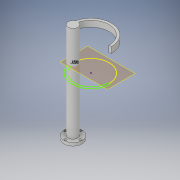
# Autodesk Inventor part: pincherleft
Saved by Autodesk Inventor 2017 (Build 210142000, 142)
## iProperties
Created: 2017-11-18
Part Number: pincherleft
Material: Generic
Document SubType Name: Modeling
Designer: User
Density: 1 g/cm^3
Appearance: Default
Author: User
Autodesk Inventor part; units mm, degrees
ref_plane "YZ Plane" through (0, 0, 0) normal (1, 0, 0) x (0, 1, 0)
ref_plane "XZ Plane" through (0, 0, 0) normal (0, 1, 0) x (-1, 0, 0)
ref_plane "XY Plane" through (0, 0, 0) normal (0, 0, 1) x (1, 0, 0)
sketch "Sketch1" plane through (0, 0, 0) normal (0, 1, 0) x (-1, 0, 0)
  circle A0 centre (0, 0) radius 5.08
  dimension "d0" = 10.16
  constraints: 1 centre point, 1 coincident
  measures "d0" diameter of A0
extrude "Extrusion1" add sketch "Sketch1" along normal blind 101.6
sketch "Sketch2" plane through (0, 101.6, 0) normal (0, 1, 0) x (1, 0, 0)
  circle A0 centre (0, 0) radius 5.08 projected
  line L0 (0, 0) -> (-2.54, 0)
  line L1 (38.1, 0) -> (40.64, 0)
  arc A1 (38.1, 0) -> (0, 0) centre (19.05, 0) ccw
  arc A2 (40.64, 0) -> (-2.54, 0) centre (19.05, 0) ccw
  line L2 (38.1, 0) -> (40.64, 0) construction
  line L3 (5.08, 0) -> (-2.54, 0) construction
  line L4 (-2.54, 0) -> (5.08, 0)
  line L5 (38.1, 0) -> (40.64, 0)
  dimension "d64" = 2.54
  dimension "d65" = 2.54
  dimension "d66" = 38.1
  dimension "d67" = 19.05
  dimension "d68" = 180
  dimension "d69" = 21.59
  constraints: 12 end point, 4 point on circle, 2 centre point, 2 coincident, 2 horizontal, 1 horizontal alignment, 1 other
  measures "d64" distance of L0.start L0.end
  measures "d65" distance of L1.start L1.end
  measures "d66" distance of L1.start L0.start
  measures "d67" distance of L1.start point (19.05, 0)
  measures "d68" angle of L3 L2
  measures "d69" distance of A2.centre L1.end
extrude "Extrusion5" add sketch "Sketch2" against normal blind 6.35 contours A1 L0 A2 A0 | A0 A2 L1 A1
sketch "Sketch4" plane through (0, 0, 0) normal (0, -1, 0) x (1, 0, 0)
  circle A0 centre (0, 0) radius 9.525
  dimension "d72" = 19.05
  constraints: 1 centre point, 1 coincident
  measures "d72" diameter of A0
extrude "Extrusion6" add sketch "Sketch4" along normal blind 3.175
sketch "Sketch5" plane through (0, -3.175, 0) normal (0, -1, 0) x (1, 0, 0)
  point P0 (0, 0)
  point P1 (0, 8.001)
  point P2 (0, -8.001)
  point P3 (8.001, 0)
  point P4 (-8.001, 0)
  dimension "d79" = 8.001
  dimension "d80" = 8.001
  dimension "d81" = 8.001
  dimension "d82" = 8.001
  measures "d79" distance of point (0, 0) point (0, 8.001)
  measures "d80" distance of point (0, 0) point (0, -8.001)
  measures "d81" distance of point (-8.001, 0) point (0, 0)
  measures "d82" distance of point (0, 0) point (8.001, 0)
hole "Hole1" at (0, -3.175, 8.001) at (0, -3.175, -8.001) at (8.001, -3.175, 0) at (-8.001, -3.175, 0) direction (0, 1, 0) diameter 2.4892 depth 25.4 tip angle 118
ref_plane "Work Plane6" through (0, 66.675, 0) normal (0, 1, 0) x (1, 0, 0)
sketch "Sketch6" plane through (0, 66.675, 0) normal (0, 1, 0) x (1, 0, 0)
  line L0 (0, 0) -> (1.27, 0)
  line L1 (1.27, 0) -> (-1.27, 0)
  arc A0 (38.1, 0) -> (0.6773, 5.0346) centre (19.05, 0) ccw projected
  arc A1 (1.27, 0) -> (36.83, 0) centre (19.05, 0) ccw
  arc A2 (-1.27, 0) -> (39.37, 0) centre (19.05, 0) ccw
  line L2 (39.37, 0) -> (36.83, 0)
  line L3 (1.27, 0) -> (-1.27, 0)
  dimension "d91" = 1.27
  dimension "d92" = 2.54
  constraints: 8 end point, 4 point on circle, 3 horizontal, 2 centre point, 2 coincident, 1 point on line
  measures "d91" distance of L0.end L0.start
  measures "d92" distance of L0.end L1.end
equation "\"d67\" = 0.5 * d66"
equation "\"d80\" = d79"
equation "\"d81\" = d79"
equation "\"d82\" = d79"
body "Solid1"
